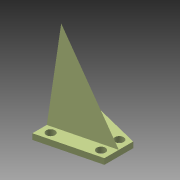
# Autodesk Inventor part: 分离前导形片
Saved by Autodesk Inventor 2015 (Build 190159000, 159)
## iProperties
Created: 2017-05-19
Part Number: 分离前导形片
Material: 常规
Document SubType Name: Modeling
Designer: Administrator
Density: 1 g/cm^3
Appearance: 铬酸锌 2
Author: Administrator
Autodesk Inventor part; units mm, degrees
ref_plane "YZ Plane" through (0, 0, 0) normal (1, 0, 0) x (0, 1, 0)
ref_plane "XZ Plane" through (0, 0, 0) normal (0, 1, 0) x (-1, 0, 0)
ref_plane "XY Plane" through (0, 0, 0) normal (0, 0, 1) x (1, 0, 0)
sketch "草图1" plane through (0, 0, 0) normal (0, 0, 1) x (1, 0, 0)
  line L0 (0, 5) -> (20, 0)
  line L1 (20, 0) -> (0, -5)
  line L2 (0, -5) -> (0, 5)
  point P0 (0, 0)
  point P1 (0, 0)
  dimension "d0" = 10
  dimension "d1" = 20
  constraints: 6 end point, 1 coincident, 1 equal length, 1 midpoint, 1 vertical
  measures "d0" distance of L1.end L0.start
  measures "d1" distance of point (0, 0) L0.end
sketch "草图2" plane through (0, 0, 0) normal (1, 0, 0) x (0, 1, 0)
  point P0 (0, 0)
  point P1 (0, 28)
  dimension "d2" = 28
  measures "d2" distance of point (0, 0) point (0, 28)
loft "放样1" add profiles "草图1" section 2 point at (0, 0, 28)
shell "抽壳1" thickness 1 removed faces 2 at (6.6667, 0, 0) at (0, 0, 9.3333)
sketch "草图3" plane through (0, 3.9539, 0) normal (0, 0, -1) x (-1, 0, 0)
  line L0 (0, -13.9539) -> (-20, -13.9539)
  line L1 (-20, -13.9539) -> (-20, 6.0461)
  line L2 (-20, 6.0461) -> (0, 6.0461)
  line L3 (0, 6.0461) -> (0, -13.9539)
  line L4 (0, -13.9539) -> (-20, -8.9539)
  line L5 (0, 6.0461) -> (-20, 1.0461)
  line L6 (-20, -3.9539) -> (0, -8.9539) projected
  line L7 (0, 1.0461) -> (-20, -3.9539) projected
  point P0 (0, -3.9539)
  point P1 (0, -3.9539)
  dimension "d8" = 20
  constraints: 12 end point, 4 parallel, 2 coincident, 2 midpoint, 2 point on line, 1 horizontal, 1 perpendicular
  measures "d8" distance of L0.end L1.end
extrude "拉伸1" add sketch "草图3" along normal blind 2 contours L4 L1 L6 L3 | L6 L7 L3 | L7 L1 L5 L3
sketch "草图4" plane through (0, 3.9539, -2) normal (0, 0, -1) x (-1, 0, 0)
  circle A0 centre (-3, -10.6269) radius 1.5
  line L0 (-20, -8.9539) -> (0, -13.9539) projected
  circle A1 centre (-17, -7.1269) radius 1.5
  circle A2 centre (-3, 2.7192) radius 1.5
  circle A3 centre (-17, -0.7808) radius 1.5
  line L1 (0, 6.0461) -> (-20, 1.0461) projected
  line L2 (-20, 1.0461) -> (-20, -8.9539) projected
  line L3 (0, -13.9539) -> (0, 6.0461) projected
  point P0 (0, -3.9539)
  dimension "d11" = 3
  dimension "d12" = 2.5
  dimension "d13" = 3
  dimension "d14" = 3
  dimension "d15" = 3
  dimension "d16" = 2.5
  dimension "d17" = 2.5
  dimension "d18" = 2.5
  dimension "d19" = 3
  dimension "d20" = 3
  dimension "d21" = 3
  dimension "d22" = 3
  constraints: 4 centre point
  measures "d11" diameter of A0
  measures "d12" distance from line of L0 A0.centre
  measures "d13" diameter of A1
  measures "d14" diameter of A2
  measures "d15" diameter of A3
  measures "d16" distance from line of L0 A1.centre
  measures "d17" distance from line of L1 A3.centre
  measures "d18" distance from line of L1 A2.centre
  measures "d19" distance from line of L2 A1.centre
  measures "d20" distance from line of A3.centre L2
  measures "d21" distance from line of L3 A0.centre
  measures "d22" distance from line of A2.centre L3
extrude "拉伸2" cut sketch "草图4" against normal through all contours A0 | A1 | A2 | A3
